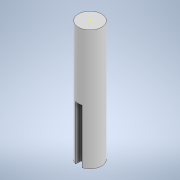
# Autodesk Inventor part: ADJ_shaft_v4
Saved by Autodesk Inventor 2022 (Build 260153000, 153)
## iProperties
Created: 2021-10-31
Part Number: ADJ_shaft_v4
Material: Generic
Document SubType Name: Modeling
Designer: shubh
Density: 1 g/cm^3
Appearance: Default
Author: shubh
Autodesk Inventor part; units mm, degrees
sketch "Sketch1" plane through (0, 0, 0) normal (0, 1, 0) x (-1, 0, 0)
  circle A0 centre (0, 0) radius 24.4517
  dimension "shaft_diameter" = 48.9034
  constraints: 1 centre point, 1 coincident
  measures "shaft_diameter" diameter of A0
extrude "Extrusion1" add sketch "Sketch1" along normal blind 254
sketch "Sketch2" plane through (0, 254, 0) normal (0, 1, 0) x (1, 0, 0)
  point P0 (0, 0)
ref_plane "Work Plane1" through (0, 247.65, 0) normal (0, 1, 0) x (1, 0, 0)
ref_plane "Work Plane2" through (0, 234.95, 0) normal (0, 1, 0) x (1, 0, 0)
sketch "Sketch6" plane through (0, 0, 0) normal (0, 0, 1) x (1, 0, 0)
  point P0 (0, 0)
ref_plane "Work Plane3" through (0, 0, 10.16) normal (0, 0, 1) x (1, 0, 0)
sketch "Sketch11" plane through (0, 0, 0) normal (0, -1, 0) x (1, 0, 0)
  circle A0 centre (0, 0) radius 24.4517 projected
  line L0 (-6.7452, 23.5029) -> (-6.7452, 12.2368)
  line L1 (-6.7452, 12.2368) -> (0, 12.2368)
  line L2 (6.7452, 23.5029) -> (6.7452, 12.2368)
  line L3 (6.7452, 12.2368) -> (0, 12.2368)
  arc A1 (6.7452, 23.5029) -> (-6.7452, 23.5029) centre (0, 0) ccw
  constraints: 8 end point, 2 point on circle, 1 centre point, 1 perpendicular, 1 vertical, 3 other
extrude "Extrusion8" cut sketch "Sketch11" against normal blind 114.3 contours L2 L3 L1 L0 A0 picked at (-4.4968, 15.9922)
body "Solid1"
